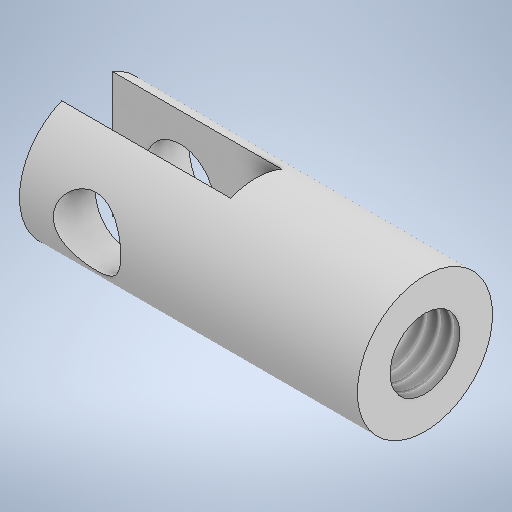
# Autodesk Inventor part: 17
Saved by Autodesk Inventor 2025.1 (Build 291241000, 241)
## iProperties
Created: 2024-09-18
Part Number: 17
Material: Generisch
Document SubType Name: Modeling
Designer: ffogue
Density: 1 g/cm^3
Appearance: Vorgabe
Author: ffogue
Autodesk Inventor part; units mm, degrees
ref_plane "YZ Plane" through (0, 0, 0) normal (1, 0, 0) x (0, 1, 0)
sketch "Sketch1" plane through (0, 0, 0) normal (0, 0, 1) x (1, 0, 0)
  line L0 (0, 0) -> (0, 4)
  line L1 (0, 4) -> (20, 4)
  line L2 (20, 4) -> (20, 0)
  line L3 (20, 0) -> (0, 0)
  dimension "d0" = 8
  dimension "d1" = 20
  constraints: 8 end point, 2 perpendicular, 1 parallel, 1 vertical
  measures "d0" diameter of L1 L3
  measures "d1" distance of L0.end L1.end
revolve "Revolution1" add sketch "Sketch1" angle 360 about axis through (20, 0, 0) along (-1, 0, 0)
ref_plane "Work Plane1" through (0, 0, 4) normal (0, 0, 1) x (1, 0, 0)
ref_plane "Work Plane3" through (0, 4, 0) normal (0, 1, 0) x (-1, 0, 0)
sketch "Sketch2" plane through (0, 0, 4) normal (0, 0, 1) x (1, 0, 0)
  line L0 (0, 4) -> (0, -4) projected
  line L1 (20, 4) -> (20, -4) projected
  line L2 (20, 4) -> (0, 4) projected
  line L3 (20, -4) -> (0, -4) projected
  line L4 (0, 1.5) -> (10, 1.5)
  line L5 (10, 1.5) -> (10, -1.5)
  line L6 (10, -1.5) -> (0, -1.5)
  line L7 (0, -1.5) -> (0, 1.5)
  point P0 (0, 0)
  point P1 (10, 0)
  point P2 (0, 0)
  point P3 (0, -1.5)
  dimension "d4" = 10
  dimension "d5" = 3
  constraints: 8 end point, 2 midpoint, 2 parallel, 1 horizontal, 1 horizontal alignment, 1 perpendicular, 1 point on line
  measures "d4" distance between parallel lines of L1 L5
  measures "d5" distance of L4.end L5.end
extrude "Extrusion1" cut sketch "Sketch2" against normal blind 8 contours L4 L5 L6 L0
sketch "Sketch4" plane through (0, 4, 0) normal (0, 1, 0) x (-1, 0, 0)
  line L0 (0, -3.7081) -> (0, 3.7081) projected
  line L1 (-20, -4) -> (-20, 4) projected
  point P0 (0, 0)
  point P1 (-4, 0)
  point P2 (0, 0)
  dimension "d18" = 16
  constraints: 1 horizontal alignment, 1 midpoint
  measures "d18" distance from line of L1 point (-4, 0)
hole "Hole2" at (4, 4, 0) direction (0, -1, 0) diameter 4 depth 8
sketch "Sketch5" plane through (20, 0, 0) normal (1, 0, 0) x (0, 0, -1)
  circle A0 centre (0, 0) radius 4 projected
  constraints: 1 coincident
hole "Hole3" at (20, 0, 0) direction (-1, 0, 0) diameter 4.134 depth 8 thread size "M5x0.8" class "6H" standard "ISO Metric profile"
body "Solid1"
